Autodesk Fusion 360 part; units mm, degrees
(part 4 of 6)
  arc A493 (59.5878, 127.7864) -> (61.8532, 128.6962) centre (60.13, 129.7115) ccw
  arc A494 (58.8286, 130.1066) -> (59.5878, 127.7864) centre (60.7139, 129.4392) ccw
  arc A495 (58.8286, 130.1066) -> (58.5606, 130.7302) centre (58.3572, 130.2734) ccw
  line L124 (58.5606, 130.7302) -> (57.9668, 130.9946)
  arc A496 (57.9668, 130.9946) -> (57.324, 130.7764) centre (57.7634, 130.5378) ccw
  arc A497 (55.0918, 129.7882) -> (57.324, 130.7764) centre (55.5665, 131.731) ccw
  arc A498 (54.2521, 132.0804) -> (55.0918, 129.7882) centre (56.1596, 131.4793) ccw
  arc A499 (54.2521, 132.0804) -> (53.9625, 132.6943) centre (53.7752, 132.2307) ccw
  line L125 (53.9625, 132.6943) -> (53.3598, 132.9378)
  arc A500 (53.3598, 132.9378) -> (52.7251, 132.6974) centre (53.1725, 132.4742) ccw
  arc A501 (50.5287, 131.6318) -> (52.7251, 132.6974) centre (50.9353, 133.59) ccw
  arc A502 (49.6095, 133.8933) -> (50.5287, 131.6318) centre (51.5368, 133.3591) ccw
  arc A503 (49.6095, 133.8933) -> (49.2987, 134.4967) centre (49.1277, 134.0269) ccw
  line L126 (49.2987, 134.4967) -> (48.6879, 134.719)
  arc A504 (48.6879, 134.719) -> (48.0619, 134.4566) centre (48.5169, 134.2492) ccw
  arc A505 (45.904, 133.315) -> (48.0619, 134.4566) centre (46.2421, 135.2862) ccw
  arc A506 (44.9065, 135.5431) -> (45.904, 133.315) centre (46.8513, 135.0765) ccw
  arc A507 (44.9065, 135.5431) -> (44.5748, 136.1353) centre (44.4203, 135.6598) ccw
  line L127 (44.5748, 136.1353) -> (43.9566, 136.3362)
  arc A508 (43.9566, 136.3362) -> (43.3402, 136.052) centre (43.8021, 135.8606) ccw
  arc A509 (41.2235, 134.8358) -> (43.3402, 136.052) centre (41.4925, 136.8177) ccw
  arc A510 (40.1487, 137.0278) -> (41.2235, 134.8358) centre (42.1086, 136.6293) ccw
  arc A511 (40.1487, 137.0278) -> (39.7966, 137.608) centre (39.6587, 137.1274) ccw
  line L128 (39.7966, 137.608) -> (39.1717, 137.7872)
  arc A512 (39.1717, 137.7872) -> (38.5656, 137.4817) centre (39.0339, 137.3065) ccw
  arc A513 (36.4926, 136.1924) -> (38.5656, 137.4817) centre (36.6924, 138.1824) ccw
  arc A514 (35.3421, 138.3455) -> (36.4926, 136.1924) centre (37.3147, 138.0156) ccw
  arc A515 (35.3421, 138.3455) -> (34.9699, 138.9131) centre (34.8489, 138.4279) ccw
  line L129 (34.9699, 138.9131) -> (34.3392, 139.0703)
  arc A516 (34.3392, 139.0703) -> (33.7441, 138.7439) centre (34.2182, 138.5852) ccw
  arc A517 (31.7174, 137.383) -> (33.7441, 138.7439) centre (31.8475, 139.3787) ccw
  arc A518 (30.4923, 139.4946) -> (31.7174, 137.383) centre (32.4753, 139.2338) ccw
  arc A519 (30.4923, 139.4946) -> (30.1006, 140.0489) centre (29.9966, 139.5598) ccw
  line L130 (30.1006, 140.0489) -> (29.4648, 140.184)
  arc A520 (29.4648, 140.184) -> (28.8814, 139.837) centre (29.3608, 139.6949) ccw
  arc A521 (26.9034, 138.4062) -> (28.8814, 139.837) centre (26.9639, 140.4053) ccw
  arc A522 (25.6055, 140.4738) -> (26.9034, 138.4062) centre (27.5963, 140.2824) ccw
  arc A523 (25.6055, 140.4738) -> (25.1946, 141.014) centre (25.1078, 140.5216) ccw
  line L131 (25.1946, 141.014) -> (24.5545, 141.1269)
  arc A524 (24.5545, 141.1269) -> (23.9836, 140.7598) centre (24.4676, 140.6345) ccw
  arc A525 (22.0567, 139.2608) -> (23.9836, 140.7598) centre (22.0474, 141.2608) ccw
  arc A526 (20.6874, 141.2818) -> (22.0567, 139.2608) centre (22.6837, 141.16) ccw
  arc A527 (20.6874, 141.2818) -> (20.2579, 141.8074) centre (20.1883, 141.3123) ccw
  line L132 (20.2579, 141.8074) -> (19.6143, 141.8979)
  arc A528 (19.6143, 141.8979) -> (19.0565, 141.511) centre (19.5447, 141.4028) ccw
  arc A529 (17.1832, 139.9458) -> (19.0565, 141.511) centre (17.104, 141.9442) ccw
  arc A530 (15.7441, 141.9177) -> (17.1832, 139.9458) centre (17.7435, 141.8657) ccw
  arc A531 (15.7441, 141.9177) -> (15.2966, 142.428) centre (15.2443, 141.9308) ccw
  line L133 (15.2966, 142.428) -> (14.6501, 142.496)
  arc A532 (14.6501, 142.496) -> (14.1063, 142.0899) centre (14.5979, 141.9987) ccw
  arc A533 (12.2887, 140.4602) -> (14.1063, 142.0899) centre (12.1398, 142.4546) ccw
  arc A534 (10.7817, 142.3808) -> (12.2887, 140.4602) centre (12.7816, 142.3985) ccw
  arc A535 (10.7817, 142.3808) -> (10.3166, 142.8751) centre (10.2817, 142.3763) ccw
  line L134 (10.3166, 142.8751) -> (9.6682, 142.9205)
  arc A536 (9.6682, 142.9205) -> (9.1388, 142.4956) centre (9.6333, 142.4217) ccw
  arc A537 (7.3792, 140.8035) -> (9.1388, 142.4956) centre (7.1608, 142.7915) ccw
  arc A538 (5.8061, 142.6703) -> (7.3792, 140.8035) centre (7.8042, 142.7578) ccw
  arc A539 (5.8061, 142.6703) -> (5.324, 143.1481) centre (5.3066, 142.6484) ccw
  line L135 (5.324, 143.1481) -> (4.6744, 143.1708)
  arc A540 (4.6744, 143.1708) -> (4.1602, 142.7278) centre (4.657, 142.6711) ccw
  arc A541 (2.4607, 140.9752) -> (4.1602, 142.7278) centre (2.1731, 142.9545) ccw
  arc A542 (0.8235, 142.786) -> (2.4607, 140.9752) centre (2.8173, 142.9432) ccw
  arc A543 (0.8235, 142.786) -> (0.325, 143.2467) centre (0.325, 142.7467) ccw
  line L136 (0.325, 143.2467) -> (-0.325, 143.2467)
  arc A544 (-0.325, 143.2467) -> (-0.8235, 142.786) centre (-0.325, 142.7467) ccw
  arc A545 (-2.4607, 140.9752) -> (-0.8235, 142.786) centre (-2.8173, 142.9432) ccw
  arc A546 (-4.1602, 142.7278) -> (-2.4607, 140.9752) centre (-2.1731, 142.9545) ccw
  arc A547 (-4.1602, 142.7278) -> (-4.6744, 143.1708) centre (-4.657, 142.6711) ccw
  line L137 (-4.6744, 143.1708) -> (-5.324, 143.1481)
  arc A548 (-5.324, 143.1481) -> (-5.8061, 142.6703) centre (-5.3066, 142.6484) ccw
  arc A549 (-7.3792, 140.8035) -> (-5.8061, 142.6703) centre (-7.8042, 142.7578) ccw
  arc A550 (-9.1388, 142.4956) -> (-7.3792, 140.8035) centre (-7.1608, 142.7915) ccw
  arc A551 (-9.1388, 142.4956) -> (-9.6682, 142.9205) centre (-9.6333, 142.4217) ccw
  line L138 (-9.6682, 142.9205) -> (-10.3166, 142.8751)
  arc A552 (-10.3166, 142.8751) -> (-10.7817, 142.3808) centre (-10.2817, 142.3763) ccw
  arc A553 (-12.2887, 140.4602) -> (-10.7817, 142.3808) centre (-12.7816, 142.3985) ccw
  arc A554 (-14.1063, 142.0899) -> (-12.2887, 140.4602) centre (-12.1398, 142.4546) ccw
  arc A555 (-14.1063, 142.0899) -> (-14.6501, 142.496) centre (-14.5979, 141.9987) ccw
  line L139 (-14.6501, 142.496) -> (-15.2966, 142.428)
  arc A556 (-15.2966, 142.428) -> (-15.7441, 141.9177) centre (-15.2443, 141.9308) ccw
  arc A557 (-17.1832, 139.9458) -> (-15.7441, 141.9177) centre (-17.7435, 141.8657) ccw
  arc A558 (-19.0565, 141.511) -> (-17.1832, 139.9458) centre (-17.104, 141.9442) ccw
  arc A559 (-19.0565, 141.511) -> (-19.6143, 141.8979) centre (-19.5447, 141.4028) ccw
  line L140 (-19.6143, 141.8979) -> (-20.2579, 141.8074)
  arc A560 (-20.2579, 141.8074) -> (-20.6874, 141.2818) centre (-20.1883, 141.3123) ccw
  arc A561 (-22.0567, 139.2608) -> (-20.6874, 141.2818) centre (-22.6837, 141.16) ccw
  arc A562 (-23.9836, 140.7598) -> (-22.0567, 139.2608) centre (-22.0474, 141.2608) ccw
  arc A563 (-23.9836, 140.7598) -> (-24.5545, 141.1269) centre (-24.4676, 140.6345) ccw
  line L141 (-24.5545, 141.1269) -> (-25.1946, 141.014)
  arc A564 (-25.1946, 141.014) -> (-25.6055, 140.4738) centre (-25.1078, 140.5216) ccw
  arc A565 (-26.9034, 138.4062) -> (-25.6055, 140.4738) centre (-27.5963, 140.2824) ccw
  arc A566 (-28.8814, 139.837) -> (-26.9034, 138.4062) centre (-26.9639, 140.4053) ccw
  arc A567 (-28.8814, 139.837) -> (-29.4648, 140.184) centre (-29.3608, 139.6949) ccw
  line L142 (-29.4648, 140.184) -> (-30.1006, 140.0489)
  arc A568 (-30.1006, 140.0489) -> (-30.4923, 139.4946) centre (-29.9966, 139.5598) ccw
  arc A569 (-31.7174, 137.383) -> (-30.4923, 139.4946) centre (-32.4753, 139.2338) ccw
  arc A570 (-33.7441, 138.7439) -> (-31.7174, 137.383) centre (-31.8475, 139.3787) ccw
  arc A571 (-33.7441, 138.7439) -> (-34.3392, 139.0703) centre (-34.2182, 138.5852) ccw
  line L143 (-34.3392, 139.0703) -> (-34.9699, 138.9131)
  arc A572 (-34.9699, 138.9131) -> (-35.3421, 138.3455) centre (-34.8489, 138.4279) ccw
  arc A573 (-36.4926, 136.1924) -> (-35.3421, 138.3455) centre (-37.3147, 138.0156) ccw
  arc A574 (-38.5656, 137.4817) -> (-36.4926, 136.1924) centre (-36.6924, 138.1824) ccw
  arc A575 (-38.5656, 137.4817) -> (-39.1717, 137.7872) centre (-39.0339, 137.3065) ccw
  line L144 (-39.1717, 137.7872) -> (-39.7966, 137.608)
  arc A576 (-39.7966, 137.608) -> (-40.1487, 137.0278) centre (-39.6587, 137.1274) ccw
  arc A577 (-41.2235, 134.8358) -> (-40.1487, 137.0278) centre (-42.1086, 136.6293) ccw
  arc A578 (-43.3402, 136.052) -> (-41.2235, 134.8358) centre (-41.4925, 136.8177) ccw
  arc A579 (-43.3402, 136.052) -> (-43.9566, 136.3362) centre (-43.8021, 135.8606) ccw
  line L145 (-43.9566, 136.3362) -> (-44.5748, 136.1353)
  arc A580 (-44.5748, 136.1353) -> (-44.9065, 135.5431) centre (-44.4203, 135.6598) ccw
  arc A581 (-45.904, 133.315) -> (-44.9065, 135.5431) centre (-46.8513, 135.0765) ccw
  arc A582 (-48.0619, 134.4566) -> (-45.904, 133.315) centre (-46.2421, 135.2862) ccw
  arc A583 (-48.0619, 134.4566) -> (-48.6879, 134.719) centre (-48.5169, 134.2492) ccw
  line L146 (-48.6879, 134.719) -> (-49.2987, 134.4967)
  arc A584 (-49.2987, 134.4967) -> (-49.6095, 133.8933) centre (-49.1277, 134.0269) ccw
  arc A585 (-50.5287, 131.6318) -> (-49.6095, 133.8933) centre (-51.5368, 133.3591) ccw
  arc A586 (-52.7251, 132.6974) -> (-50.5287, 131.6318) centre (-50.9353, 133.59) ccw
  arc A587 (-52.7251, 132.6974) -> (-53.3598, 132.9378) centre (-53.1725, 132.4742) ccw
  line L147 (-53.3598, 132.9378) -> (-53.9625, 132.6943)
  arc A588 (-53.9625, 132.6943) -> (-54.2521, 132.0804) centre (-53.7752, 132.2307) ccw
  arc A589 (-55.0918, 129.7882) -> (-54.2521, 132.0804) centre (-56.1596, 131.4793) ccw
  arc A590 (-57.324, 130.7764) -> (-55.0918, 129.7882) centre (-55.5665, 131.731) ccw
  arc A591 (-57.324, 130.7764) -> (-57.9668, 130.9946) centre (-57.7634, 130.5378) ccw
  line L148 (-57.9668, 130.9946) -> (-58.5606, 130.7302)
  arc A592 (-58.5606, 130.7302) -> (-58.8286, 130.1066) centre (-58.3572, 130.2734) ccw
  arc A593 (-59.5878, 127.7864) -> (-58.8286, 130.1066) centre (-60.7139, 129.4392) ccw
  arc A594 (-61.8532, 128.6962) -> (-59.5878, 127.7864) centre (-60.13, 129.7115) ccw
  arc A595 (-61.8532, 128.6962) -> (-62.5031, 128.8918) centre (-62.2839, 128.4424) ccw
  line L149 (-62.5031, 128.8918) -> (-63.0873, 128.6068)
  arc A596 (-63.0873, 128.6068) -> (-63.3334, 127.9742) centre (-62.8682, 128.1574) ccw
  arc A597 (-64.0112, 125.629) -> (-63.3334, 127.9742) centre (-65.1943, 127.2415) ccw
  arc A598 (-66.3069, 126.4592) -> (-64.0112, 125.629) centre (-64.6203, 127.534) ccw
  arc A599 (-66.3069, 126.4592) -> (-66.9633, 126.6319) centre (-66.7286, 126.1905) ccw
  line L150 (-66.9633, 126.6319) -> (-67.5372, 126.3268)
  arc A600 (-67.5372, 126.3268) -> (-67.761, 125.686) centre (-67.3025, 125.8853) ccw
  arc A601 (-68.3566, 123.3185) -> (-67.761, 125.686) centre (-69.5953, 124.8887) ccw
  arc A602 (-70.6799, 124.068) -> (-68.3566, 123.3185) centre (-69.0318, 125.2011) ccw
  arc A603 (-70.6799, 124.068) -> (-71.3419, 124.2178) centre (-71.0919, 123.7848) ccw
  line L151 (-71.3419, 124.2178) -> (-71.9048, 123.8928)
  arc A604 (-71.9048, 123.8928) -> (-72.1061, 123.2446) centre (-71.6548, 123.4598) ccw
  arc A605 (-72.6187, 120.8578) -> (-72.1061, 123.2446) centre (-73.9114, 122.3838) ccw
  arc A606 (-74.9667, 121.5258) -> (-72.6187, 120.8578) centre (-73.3592, 122.7156) ccw
  arc A607 (-74.9667, 121.5258) -> (-75.6336, 121.6523) centre (-75.3686, 121.2283) ccw
  line L152 (-75.6336, 121.6523) -> (-76.1848, 121.3079)
  arc A608 (-76.1848, 121.3079) -> (-76.3634, 120.653) centre (-75.9199, 120.8839) ccw
  arc A609 (-76.7923, 118.2498) -> (-76.3634, 120.653) centre (-78.1375, 119.7298) ccw
  arc A610 (-79.1623, 118.8354) -> (-76.7923, 118.2498) centre (-77.5972, 120.0807) ccw
  arc A611 (-79.1623, 118.8354) -> (-79.8331, 118.9387) centre (-79.5535, 118.5241) ccw
  line L153 (-79.8331, 118.9387) -> (-80.372, 118.5752)
  arc A612 (-80.372, 118.5752) -> (-80.5276, 117.9145) centre (-80.0924, 118.1607) ccw
  arc A613 (-80.8724, 115.4978) -> (-80.5276, 117.9145) centre (-82.2684, 116.9299) ccw
  arc A614 (-83.2613, 116.0003) -> (-80.8724, 115.4978) centre (-81.7407, 117.2994) ccw
  arc A615 (-83.2613, 116.0003) -> (-83.9354, 116.0801) centre (-83.6415, 115.6756) ccw
  line L154 (-83.9354, 116.0801) -> (-84.4612, 115.698)
  arc A616 (-84.4612, 115.698) -> (-84.5937, 115.0323) centre (-84.1673, 115.2935) ccw
  arc A617 (-84.8539, 112.605) -> (-84.5937, 115.0323) centre (-86.2991, 113.9875) ccw
  arc A618 (-87.259, 113.0239) -> (-84.8539, 112.605) centre (-85.7846, 114.3753) ccw
  arc A619 (-87.259, 113.0239) -> (-87.9354, 113.08) centre (-87.6276, 112.686) ccw
  line L155 (-87.9354, 113.08) -> (-88.4476, 112.6799)
  arc A620 (-88.4476, 112.6799) -> (-88.5567, 112.01) centre (-88.1398, 112.2859) ccw
  arc A621 (-88.7321, 109.575) -> (-88.5567, 112.01) centre (-90.2247, 110.9063) ccw
  arc A622 (-91.1503, 109.9097) -> (-88.7321, 109.575) centre (-89.724, 111.3118) ccw
  arc A623 (-91.1503, 109.9097) -> (-91.8283, 109.9423) centre (-91.5069, 109.5592) ccw
  line L156 (-91.8283, 109.9423) -> (-92.3262, 109.5244)
  arc A624 (-92.3262, 109.5244) -> (-92.4119, 108.8511) centre (-92.0048, 109.1414) ccw
  arc A625 (-92.5022, 106.4116) -> (-92.4119, 108.8511) centre (-94.0403, 107.6899) ccw
  arc A626 (-94.9306, 106.6617) -> (-92.5022, 106.4116) centre (-93.554, 108.1126) ccw
  arc A627 (-94.9306, 106.6617) -> (-95.6092, 106.6705) centre (-95.2747, 106.299) ccw
  line L157 (-95.6092, 106.6705) -> (-96.0923, 106.2356)
  arc A628 (-96.0923, 106.2356) -> (-96.1544, 105.5597) centre (-95.7577, 105.864) ccw
  arc A629 (-96.1595, 103.1185) -> (-96.1544, 105.5597) centre (-97.7413, 104.3424) ccw
  arc A630 (-98.5952, 103.2837) -> (-96.1595, 103.1185) centre (-97.2701, 104.7818) ccw
  arc A631 (-98.5952, 103.2837) -> (-99.2737, 103.2688) centre (-98.9264, 102.9092) ccw
  line L158 (-99.2737, 103.2688) -> (-99.7413, 102.8173)
  arc A632 (-99.7413, 102.8173) -> (-99.7798, 102.1396) centre (-99.394, 102.4576) ccw
  arc A633 (-99.6997, 99.6997) -> (-99.7798, 102.1396) centre (-101.3233, 100.8677) ccw
  arc A634 (-102.1396, 99.7798) -> (-99.6997, 99.6997) centre (-100.8677, 101.3233) ccw
  arc A635 (-102.1396, 99.7798) -> (-102.8173, 99.7413) centre (-102.4576, 99.394) ccw
  line L159 (-102.8173, 99.7413) -> (-103.2688, 99.2737)
  arc A636 (-103.2688, 99.2737) -> (-103.2837, 98.5952) centre (-102.9092, 98.9264) ccw
  arc A637 (-103.1185, 96.1595) -> (-103.2837, 98.5952) centre (-104.7818, 97.2701) ccw
  arc A638 (-105.5597, 96.1544) -> (-103.1185, 96.1595) centre (-104.3424, 97.7413) ccw
  arc A639 (-105.5597, 96.1544) -> (-106.2356, 96.0923) centre (-105.864, 95.7577) ccw
  line L160 (-106.2356, 96.0923) -> (-106.6705, 95.6092)
  arc A640 (-106.6705, 95.6092) -> (-106.6617, 94.9306) centre (-106.299, 95.2747) ccw
  arc A641 (-106.4116, 92.5022) -> (-106.6617, 94.9306) centre (-108.1126, 93.554) ccw
  arc A642 (-108.8511, 92.4119) -> (-106.4116, 92.5022) centre (-107.6899, 94.0403) ccw
  arc A643 (-108.8511, 92.4119) -> (-109.5244, 92.3262) centre (-109.1414, 92.0048) ccw
  line L161 (-109.5244, 92.3262) -> (-109.9423, 91.8283)
  arc A644 (-109.9423, 91.8283) -> (-109.9097, 91.1503) centre (-109.5592, 91.5069) ccw
  arc A645 (-109.575, 88.7321) -> (-109.9097, 91.1503) centre (-111.3118, 89.724) ccw
  arc A646 (-112.01, 88.5567) -> (-109.575, 88.7321) centre (-110.9063, 90.2247) ccw
  arc A647 (-112.01, 88.5567) -> (-112.6799, 88.4476) centre (-112.2859, 88.1398) ccw
  line L162 (-112.6799, 88.4476) -> (-113.08, 87.9354)
  arc A648 (-113.08, 87.9354) -> (-113.0239, 87.259) centre (-112.686, 87.6276) ccw
  arc A649 (-112.605, 84.8539) -> (-113.0239, 87.259) centre (-114.3753, 85.7846) ccw
  arc A650 (-115.0323, 84.5937) -> (-112.605, 84.8539) centre (-113.9875, 86.2991) ccw
  arc A651 (-115.0323, 84.5937) -> (-115.698, 84.4612) centre (-115.2935, 84.1673) ccw
  line L163 (-115.698, 84.4612) -> (-116.0801, 83.9354)
  arc A652 (-116.0801, 83.9354) -> (-116.0003, 83.2613) centre (-115.6756, 83.6415) ccw
  arc A653 (-115.4978, 80.8724) -> (-116.0003, 83.2613) centre (-117.2994, 81.7407) ccw
  arc A654 (-117.9145, 80.5276) -> (-115.4978, 80.8724) centre (-116.9299, 82.2684) ccw
  arc A655 (-117.9145, 80.5276) -> (-118.5752, 80.372) centre (-118.1607, 80.0924) ccw
  line L164 (-118.5752, 80.372) -> (-118.9387, 79.8331)
  arc A656 (-118.9387, 79.8331) -> (-118.8354, 79.1623) centre (-118.5241, 79.5535) ccw
  arc A657 (-118.2498, 76.7923) -> (-118.8354, 79.1623) centre (-120.0807, 77.5972) ccw
  arc A658 (-120.653, 76.3634) -> (-118.2498, 76.7923) centre (-119.7298, 78.1375) ccw
  arc A659 (-120.653, 76.3634) -> (-121.3079, 76.1848) centre (-120.8839, 75.9199) ccw
  line L165 (-121.3079, 76.1848) -> (-121.6523, 75.6336)
  arc A660 (-121.6523, 75.6336) -> (-121.5258, 74.9667) centre (-121.2283, 75.3686) ccw
  arc A661 (-120.8578, 72.6187) -> (-121.5258, 74.9667) centre (-122.7156, 73.3592) ccw
  arc A662 (-123.2446, 72.1061) -> (-120.8578, 72.6187) centre (-122.3838, 73.9114) ccw
  arc A663 (-123.2446, 72.1061) -> (-123.8928, 71.9048) centre (-123.4598, 71.6548) ccw
  line L166 (-123.8928, 71.9048) -> (-124.2178, 71.3419)
  arc A664 (-124.2178, 71.3419) -> (-124.068, 70.6799) centre (-123.7848, 71.0919) ccw
  arc A665 (-123.3185, 68.3566) -> (-124.068, 70.6799) centre (-125.2011, 69.0318) ccw
  arc A666 (-125.686, 67.761) -> (-123.3185, 68.3566) centre (-124.8887, 69.5953) ccw
  arc A667 (-125.686, 67.761) -> (-126.3268, 67.5372) centre (-125.8853, 67.3025) ccw
  line L167 (-126.3268, 67.5372) -> (-126.6319, 66.9633)
  arc A668 (-126.6319, 66.9633) -> (-126.4592, 66.3069) centre (-126.1905, 66.7286) ccw
  arc A669 (-125.629, 64.0112) -> (-126.4592, 66.3069) centre (-127.534, 64.6203) ccw
  arc A670 (-127.9742, 63.3334) -> (-125.629, 64.0112) centre (-127.2415, 65.1943) ccw
  arc A671 (-127.9742, 63.3334) -> (-128.6068, 63.0873) centre (-128.1574, 62.8682) ccw
  line L168 (-128.6068, 63.0873) -> (-128.8918, 62.5031)
  arc A672 (-128.8918, 62.5031) -> (-128.6962, 61.8532) centre (-128.4424, 62.2839) ccw
  arc A673 (-127.7864, 59.5878) -> (-128.6962, 61.8532) centre (-129.7115, 60.13) ccw
  arc A674 (-130.1066, 58.8286) -> (-127.7864, 59.5878) centre (-129.4392, 60.7139) ccw
  arc A675 (-130.1066, 58.8286) -> (-130.7302, 58.5606) centre (-130.2734, 58.3572) ccw
  line L169 (-130.7302, 58.5606) -> (-130.9946, 57.9668)
  arc A676 (-130.9946, 57.9668) -> (-130.7764, 57.324) centre (-130.5378, 57.7634) ccw
  arc A677 (-129.7882, 55.0918) -> (-130.7764, 57.324) centre (-131.731, 55.5665) ccw
  arc A678 (-132.0804, 54.2521) -> (-129.7882, 55.0918) centre (-131.4793, 56.1596) ccw
  arc A679 (-132.0804, 54.2521) -> (-132.6943, 53.9625) centre (-132.2307, 53.7752) ccw
  line L170 (-132.6943, 53.9625) -> (-132.9378, 53.3598)
  arc A680 (-132.9378, 53.3598) -> (-132.6974, 52.7251) centre (-132.4742, 53.1725) ccw
  arc A681 (-131.6318, 50.5287) -> (-132.6974, 52.7251) centre (-133.59, 50.9353) ccw
  arc A682 (-133.8933, 49.6095) -> (-131.6318, 50.5287) centre (-133.3591, 51.5368) ccw
  arc A683 (-133.8933, 49.6095) -> (-134.4967, 49.2987) centre (-134.0269, 49.1277) ccw
  line L171 (-134.4967, 49.2987) -> (-134.719, 48.6879)
  arc A684 (-134.719, 48.6879) -> (-134.4566, 48.0619) centre (-134.2492, 48.5169) ccw
  arc A685 (-133.315, 45.904) -> (-134.4566, 48.0619) centre (-135.2862, 46.2421) ccw
  arc A686 (-135.5431, 44.9065) -> (-133.315, 45.904) centre (-135.0765, 46.8513) ccw
  arc A687 (-135.5431, 44.9065) -> (-136.1353, 44.5748) centre (-135.6598, 44.4203) ccw
  line L172 (-136.1353, 44.5748) -> (-136.3362, 43.9566)
  arc A688 (-136.3362, 43.9566) -> (-136.052, 43.3402) centre (-135.8606, 43.8021) ccw
  arc A689 (-134.8358, 41.2235) -> (-136.052, 43.3402) centre (-136.8177, 41.4925) ccw
  arc A690 (-137.0278, 40.1487) -> (-134.8358, 41.2235) centre (-136.6293, 42.1086) ccw
  arc A691 (-137.0278, 40.1487) -> (-137.608, 39.7966) centre (-137.1274, 39.6587) ccw
  line L173 (-137.608, 39.7966) -> (-137.7872, 39.1717)
  arc A692 (-137.7872, 39.1717) -> (-137.4817, 38.5656) centre (-137.3065, 39.0339) ccw
  arc A693 (-136.1924, 36.4926) -> (-137.4817, 38.5656) centre (-138.1824, 36.6924) ccw
  arc A694 (-138.3455, 35.3421) -> (-136.1924, 36.4926) centre (-138.0156, 37.3147) ccw
  arc A695 (-138.3455, 35.3421) -> (-138.9131, 34.9699) centre (-138.4279, 34.8489) ccw
  line L174 (-138.9131, 34.9699) -> (-139.0703, 34.3392)
  arc A696 (-139.0703, 34.3392) -> (-138.7439, 33.7441) centre (-138.5852, 34.2182) ccw
  arc A697 (-137.383, 31.7174) -> (-138.7439, 33.7441) centre (-139.3787, 31.8475) ccw
  arc A698 (-139.4946, 30.4923) -> (-137.383, 31.7174) centre (-139.2338, 32.4753) ccw
  arc A699 (-139.4946, 30.4923) -> (-140.0489, 30.1006) centre (-139.5598, 29.9966) ccw
  line L175 (-140.0489, 30.1006) -> (-140.184, 29.4648)
  arc A700 (-140.184, 29.4648) -> (-139.837, 28.8814) centre (-139.6949, 29.3608) ccw
  arc A701 (-138.4062, 26.9034) -> (-139.837, 28.8814) centre (-140.4053, 26.9639) ccw
  arc A702 (-140.4738, 25.6055) -> (-138.4062, 26.9034) centre (-140.2824, 27.5963) ccw
  arc A703 (-140.4738, 25.6055) -> (-141.014, 25.1946) centre (-140.5216, 25.1078) ccw
  line L176 (-141.014, 25.1946) -> (-141.1269, 24.5545)
  arc A704 (-141.1269, 24.5545) -> (-140.7598, 23.9836) centre (-140.6345, 24.4676) ccw
  arc A705 (-139.2608, 22.0567) -> (-140.7598, 23.9836) centre (-141.2608, 22.0474) ccw
  arc A706 (-141.2818, 20.6874) -> (-139.2608, 22.0567) centre (-141.16, 22.6837) ccw
  arc A707 (-141.2818, 20.6874) -> (-141.8074, 20.2579) centre (-141.3123, 20.1883) ccw
  line L177 (-141.8074, 20.2579) -> (-141.8979, 19.6143)
  arc A708 (-141.8979, 19.6143) -> (-141.511, 19.0565) centre (-141.4028, 19.5447) ccw
  arc A709 (-139.9458, 17.1832) -> (-141.511, 19.0565) centre (-141.9442, 17.104) ccw
  arc A710 (-141.9177, 15.7441) -> (-139.9458, 17.1832) centre (-141.8657, 17.7435) ccw
  arc A711 (-141.9177, 15.7441) -> (-142.428, 15.2966) centre (-141.9308, 15.2443) ccw
  line L178 (-142.428, 15.2966) -> (-142.496, 14.6501)
  arc A712 (-142.496, 14.6501) -> (-142.0899, 14.1063) centre (-141.9987, 14.5979) ccw
  arc A713 (-140.4602, 12.2887) -> (-142.0899, 14.1063) centre (-142.4546, 12.1398) ccw
  arc A714 (-142.3808, 10.7817) -> (-140.4602, 12.2887) centre (-142.3985, 12.7816) ccw
  arc A715 (-142.3808, 10.7817) -> (-142.8751, 10.3166) centre (-142.3763, 10.2817) ccw
  line L179 (-142.8751, 10.3166) -> (-142.9205, 9.6682)
  arc A716 (-142.9205, 9.6682) -> (-142.4956, 9.1388) centre (-142.4217, 9.6333) ccw
  arc A717 (-140.8035, 7.3792) -> (-142.4956, 9.1388) centre (-142.7915, 7.1608) ccw
  arc A718 (-142.6703, 5.8061) -> (-140.8035, 7.3792) centre (-142.7578, 7.8042) ccw
  arc A719 (-142.6703, 5.8061) -> (-143.1481, 5.324) centre (-142.6484, 5.3066) ccw
  circle A720 centre (0, 0) radius 145
  dimension "d12" = 290
  constraint coincident A720.centre origin
  measures "d12" diameter of A720
extrude "Extrude2" add sketch "Sketch2" along normal blind 2 contours L0 A0 A1 A2 A3 L1 A4 A5 A6 A7 L2 A8 A9 A10 A11 L3 A12 A13 A14 A15 L4 A16 A17 A18 A19 L5 A20 A21 A22 A23 L6 A24 A25 A26 A27 L7 A28 A29 A30 A31 L8 A32 A33 A34 A35 L9 A36 A37 A38 A39 L10 A40 A41 A42 A43 L11 A44 A45 A46 A47 L12 A48 A49 A50 A51 L13 A52 A53 A54 A55 L14 A56 A57 A58 A59 L15 A60 A61 A62 A63 L16 A64 A65 A66 A67 L17 A68 A69 A70 A71 L18 A72 A73 A74 A75 L19 A76 A77 A78 A79 L20 A80 A81 A82 A83 L21 A84 A85 A86 A87 L22 A88 A89 A90 A91 L23 A92 A93 A94 A95 L24 A96 A97 A98 A99 L25 A100 A101 A102 A103 L26 A104 A105 A106 A107 L27 A108 A109 A110 A111 L28 A112 A113 A114 A115 L29 A116 A117 A118 A119 L30 A120 A121 A122 A123 L31 A124 A125 A126 A127 L32 A128 A129 A130 A131 L33 A132 A133 A134 A135 L34 A136 A137 A138 A139 L35 A140 A141 A142 A143 L36 A144 A145 A146 A147 L37 A148 A149 A150 A151 L38 A152 A153 A154 A155 L39 A156 A157 A158 A159 L40 A160 A161 A162 A163 L41 A164 A165 A166 A167 L42 A168 A169 A170 A171 L43 A172 A173 A174 A175 L44 A176 A177 A178 A179 L45 A180 A181 A182 A183 L46 A184 A185 A186 A187 L47 A188 A189 A190 A191 L48 A192 A193 A194 A195 L49 A196 A197 A198 A199 L50 A200 A201 A202 A203 L51 A204 A205 A206 A207 L52 A208 A209 A210 A211 L53 A212 A213 A214 A215 L54 A216 A217 A218 A219 L55 A220 A221 A222 A223 L56 A224 A225 A226 A227 L57 A228 A229 A230 A231 L58 A232 A233 A234 A235 L59 A236 A237 A238 A239 L60 A240 A241 A242 A243 L61 A244 A245 A246 A247 L62 A248 A249 A250 A251 L63 A252 A253 A254 A255 L64 A256 A257 A258 A259 L65 A260 A261 A262 A263 L66 A264 A265 A266 A267 L67 A268 A269 A270 A271 L68 A272 A273 A274 A275 L69 A276 A277 A278 A279 L70 A280 A281 A282 A283 L71 A284 A285 A286 A287 L72 A288 A289 A290 A291 L73 A292 A293 A294 A295 L74 A296 A297 A298 A299 L75 A300 A301 A302 A303 L76 A304 A305 A306 A307 L77 A308 A309 A310 A311 L78 A312 A313 A314 A315 L79 A316 A317 A318 A319 L80 A320 A321 A322 A323 L81 A324 A325 A326 A327 L82 A328 A329 A330 A331 L83 A332 A333 A334 A335 L84 A336 A337 A338 A339 L85 A340 A341 A342 A343 L86 A344 A345 A346 A347 L87 A348 A349 A350 A351 L88 A352 A353 A354 A355 L89 A356 A357 A358 A359 L90 A360 A361 A362 A363 L91 A364 A365 A366 A367 L92 A368 A369 A370 A371 L93 A372 A373 A374 A375 L94 A376 A377 A378 A379 L95 A380 A381 A382 A383 L96 A384 A385 A386 A387 L97 A388 A389 A390 A391 L98 A392 A393 A394 A395 L99 A396 A397 A398 A399 L100 A400 A401 A402 A403 L101 A404 A405 A406 A407 L102 A408 A409 A410 A411 L103 A412 A413 A414 A415 L104 A416 A417 A418 A419 L105 A420 A421 A422 A423 L106 A424 A425 A426 A427 L107 A428 A429 A430 A431 L108 A432 A433 A434 A435 L109 A436 A437 A438 A439 L110 A440 A441 A442 A443 L111 A444 A445 A446 A447 L112 A448 A449 A450 A451 L113 A452 A453 A454 A455 L114 A456 A457 A458 A459 L115 A460 A461 A462 A463 L116 A464 A465 A466 A467 L117 A468 A469 A470 A471 L118 A472 A473 A474 A475 L119 A476 A477 A478 A479 L120 A480 A481 A482 A483 L121 A484 A485 A486 A487 L122 A488 A489 A490 A491 L123 A492 A493 A494 A495 L124 A496 A497 A498 A499 L125 A500 A501 A502 A503 L126 A504 A505 A506 A507 L127 A508 A509 A510 A511 L128 A512 A513 A514 A515 L129 A516 A517 A518 A519 L130 A520 A521 A522 A523 L131 A524 A525 A526 A527 L132 A528 A529 A530 A531 L133 A532 A533 A534 A535 L134 A536 A537 A538 A539 L135 A540 A541 A542 A543 L136 A544 A545 A546 A547 L137 A548 A549 A550 A551 L138 A552 A553 A554 A555 L139 A556 A557 A558 A559 L140 A560 A561 A562 A563 L141 A564 A565 A566 A567 L142 A568 A569 A570 A571 L143 A572 A573 A574 A575 L144 A576 A577 A578 A579 L145 A580 A581 A582 A583 L146 A584 A585 A586 A587 L147 A588 A589 A590 A591 L148 A592 A593 A594 A595 L149 A596 A597 A598 A599 L150 A600 A601 A602 A603 L151 A604 A605 A606 A607 L152 A608 A609 A610 A611 L153 A612 A613 A614 A615 L154 A616 A617 A618 A619 L155 A620 A621 A622 A623 L156 A624 A625 A626 A627 L157 A628 A629 A630 A631 L158 A632 A633 A634 A635 L159 A636 A637 A638 A639 L160 A640 A641 A642 A643 L161 A644 A645 A646 A647 L162 A648 A649 A650 A651 L163 A652 A653 A654 A655 L164 A656 A657 A658 A659 L165 A660 A661 A662 A663 L166 A664 A665 A666 A667 L167 A668 A669 A670 A671 L168 A672 A673 A674 A675 L169 A676 A677 A678 A679 L170 A680 A681 A682 A683 L171 A684 A685 A686 A687 L172 A688 A689 A690 A691 L173 A692 A693 A694 A695 L174 A696 A697 A698 A699 L175 A700 A701 A702 A703 L176 A704 A705 A706 A707 L177 A708 A709 A710 A711 L178 A712 A713 A714 A715 L179 A716 A717 A718 A719 | A720
sketch "Sketch3" plane through (0, 0, 0) normal (0, 0, -1) x (1, 0, 0)
  line L0 (143.1708, 4.6744) -> (143.1481, 5.324)
  arc A0 (143.1481, 5.324) -> (142.6703, 5.8061) centre (142.6484, 5.3066) ccw
  arc A1 (140.8035, 7.3792) -> (142.6703, 5.8061) centre (142.7578, 7.8042) ccw
  arc A2 (142.4956, 9.1388) -> (140.8035, 7.3792) centre (142.7915, 7.1608) ccw
  arc A3 (142.4956, 9.1388) -> (142.9205, 9.6682) centre (142.4217, 9.6333) ccw
  line L1 (142.9205, 9.6682) -> (142.8751, 10.3166)
  arc A4 (142.8751, 10.3166) -> (142.3808, 10.7817) centre (142.3763, 10.2817) ccw
  arc A5 (140.4602, 12.2887) -> (142.3808, 10.7817) centre (142.3985, 12.7816) ccw
  arc A6 (142.0899, 14.1063) -> (140.4602, 12.2887) centre (142.4546, 12.1398) ccw
  arc A7 (142.0899, 14.1063) -> (142.496, 14.6501) centre (141.9987, 14.5979) ccw
  line L2 (142.496, 14.6501) -> (142.428, 15.2966)
  arc A8 (142.428, 15.2966) -> (141.9177, 15.7441) centre (141.9308, 15.2443) ccw
  arc A9 (139.9458, 17.1832) -> (141.9177, 15.7441) centre (141.8657, 17.7435) ccw
  arc A10 (141.511, 19.0565) -> (139.9458, 17.1832) centre (141.9442, 17.104) ccw
  arc A11 (141.511, 19.0565) -> (141.8979, 19.6143) centre (141.4028, 19.5447) ccw
  line L3 (141.8979, 19.6143) -> (141.8074, 20.2579)
  arc A12 (141.8074, 20.2579) -> (141.2818, 20.6874) centre (141.3123, 20.1883) ccw
  arc A13 (139.2608, 22.0567) -> (141.2818, 20.6874) centre (141.16, 22.6837) ccw
  arc A14 (140.7598, 23.9836) -> (139.2608, 22.0567) centre (141.2608, 22.0474) ccw
  arc A15 (140.7598, 23.9836) -> (141.1269, 24.5545) centre (140.6345, 24.4676) ccw
  line L4 (141.1269, 24.5545) -> (141.014, 25.1946)
  arc A16 (141.014, 25.1946) -> (140.4738, 25.6055) centre (140.5216, 25.1078) ccw
  arc A17 (138.4062, 26.9034) -> (140.4738, 25.6055) centre (140.2824, 27.5963) ccw
  arc A18 (139.837, 28.8814) -> (138.4062, 26.9034) centre (140.4053, 26.9639) ccw
  arc A19 (139.837, 28.8814) -> (140.184, 29.4648) centre (139.6949, 29.3608) ccw
  line L5 (140.184, 29.4648) -> (140.0489, 30.1006)
  arc A20 (140.0489, 30.1006) -> (139.4946, 30.4923) centre (139.5598, 29.9966) ccw
  arc A21 (137.383, 31.7174) -> (139.4946, 30.4923) centre (139.2338, 32.4753) ccw
  arc A22 (138.7439, 33.7441) -> (137.383, 31.7174) centre (139.3787, 31.8475) ccw
  arc A23 (138.7439, 33.7441) -> (139.0703, 34.3392) centre (138.5852, 34.2182) ccw
  line L6 (139.0703, 34.3392) -> (138.9131, 34.9699)
  arc A24 (138.9131, 34.9699) -> (138.3455, 35.3421) centre (138.4279, 34.8489) ccw
  arc A25 (136.1924, 36.4926) -> (138.3455, 35.3421) centre (138.0156, 37.3147) ccw
  arc A26 (137.4817, 38.5656) -> (136.1924, 36.4926) centre (138.1824, 36.6924) ccw
  arc A27 (137.4817, 38.5656) -> (137.7872, 39.1717) centre (137.3065, 39.0339) ccw
  line L7 (137.7872, 39.1717) -> (137.608, 39.7966)
  arc A28 (137.608, 39.7966) -> (137.0278, 40.1487) centre (137.1274, 39.6587) ccw
  arc A29 (134.8358, 41.2235) -> (137.0278, 40.1487) centre (136.6293, 42.1086) ccw
  arc A30 (136.052, 43.3402) -> (134.8358, 41.2235) centre (136.8177, 41.4925) ccw
  arc A31 (136.052, 43.3402) -> (136.3362, 43.9566) centre (135.8606, 43.8021) ccw
  line L8 (136.3362, 43.9566) -> (136.1353, 44.5748)
  arc A32 (136.1353, 44.5748) -> (135.5431, 44.9065) centre (135.6598, 44.4203) ccw
  arc A33 (133.315, 45.904) -> (135.5431, 44.9065) centre (135.0765, 46.8513) ccw
  arc A34 (134.4566, 48.0619) -> (133.315, 45.904) centre (135.2862, 46.2421) ccw
  arc A35 (134.4566, 48.0619) -> (134.719, 48.6879) centre (134.2492, 48.5169) ccw
  line L9 (134.719, 48.6879) -> (134.4967, 49.2987)
  arc A36 (134.4967, 49.2987) -> (133.8933, 49.6095) centre (134.0269, 49.1277) ccw
  arc A37 (131.6318, 50.5287) -> (133.8933, 49.6095) centre (133.3591, 51.5368) ccw
  arc A38 (132.6974, 52.7251) -> (131.6318, 50.5287) centre (133.59, 50.9353) ccw
  arc A39 (132.6974, 52.7251) -> (132.9378, 53.3598) centre (132.4742, 53.1725) ccw
  line L10 (132.9378, 53.3598) -> (132.6943, 53.9625)
  arc A40 (132.6943, 53.9625) -> (132.0804, 54.2521) centre (132.2307, 53.7752) ccw
  arc A41 (129.7882, 55.0918) -> (132.0804, 54.2521) centre (131.4793, 56.1596) ccw
  arc A42 (130.7764, 57.324) -> (129.7882, 55.0918) centre (131.731, 55.5665) ccw
  arc A43 (130.7764, 57.324) -> (130.9946, 57.9668) centre (130.5378, 57.7634) ccw
  line L11 (130.9946, 57.9668) -> (130.7302, 58.5606)
  arc A44 (130.7302, 58.5606) -> (130.1066, 58.8286) centre (130.2734, 58.3572) ccw
  arc A45 (127.7864, 59.5878) -> (130.1066, 58.8286) centre (129.4392, 60.7139) ccw
  arc A46 (128.6962, 61.8532) -> (127.7864, 59.5878) centre (129.7115, 60.13) ccw
  arc A47 (128.6962, 61.8532) -> (128.8918, 62.5031) centre (128.4424, 62.2839) ccw
  line L12 (128.8918, 62.5031) -> (128.6068, 63.0873)
  arc A48 (128.6068, 63.0873) -> (127.9742, 63.3334) centre (128.1574, 62.8682) ccw
  arc A49 (125.629, 64.0112) -> (127.9742, 63.3334) centre (127.2415, 65.1943) ccw
  arc A50 (126.4592, 66.3069) -> (125.629, 64.0112) centre (127.534, 64.6203) ccw
  arc A51 (126.4592, 66.3069) -> (126.6319, 66.9633) centre (126.1905, 66.7286) ccw
  line L13 (126.6319, 66.9633) -> (126.3268, 67.5372)
  arc A52 (126.3268, 67.5372) -> (125.686, 67.761) centre (125.8853, 67.3025) ccw
  arc A53 (123.3185, 68.3566) -> (125.686, 67.761) centre (124.8887, 69.5953) ccw
  arc A54 (124.068, 70.6799) -> (123.3185, 68.3566) centre (125.2011, 69.0318) ccw
  arc A55 (124.068, 70.6799) -> (124.2178, 71.3419) centre (123.7848, 71.0919) ccw
  line L14 (124.2178, 71.3419) -> (123.8928, 71.9048)
  arc A56 (123.8928, 71.9048) -> (123.2446, 72.1061) centre (123.4598, 71.6548) ccw
  arc A57 (120.8578, 72.6187) -> (123.2446, 72.1061) centre (122.3838, 73.9114) ccw
  arc A58 (121.5258, 74.9667) -> (120.8578, 72.6187) centre (122.7156, 73.3592) ccw
  arc A59 (121.5258, 74.9667) -> (121.6523, 75.6336) centre (121.2283, 75.3686) ccw
  line L15 (121.6523, 75.6336) -> (121.3079, 76.1848)
  arc A60 (121.3079, 76.1848) -> (120.653, 76.3634) centre (120.8839, 75.9199) ccw
  arc A61 (118.2498, 76.7923) -> (120.653, 76.3634) centre (119.7298, 78.1375) ccw
  arc A62 (118.8354, 79.1623) -> (118.2498, 76.7923) centre (120.0807, 77.5972) ccw
  arc A63 (118.8354, 79.1623) -> (118.9387, 79.8331) centre (118.5241, 79.5535) ccw
  line L16 (118.9387, 79.8331) -> (118.5752, 80.372)
  arc A64 (118.5752, 80.372) -> (117.9145, 80.5276) centre (118.1607, 80.0924) ccw
  arc A65 (115.4978, 80.8724) -> (117.9145, 80.5276) centre (116.9299, 82.2684) ccw
  arc A66 (116.0003, 83.2613) -> (115.4978, 80.8724) centre (117.2994, 81.7407) ccw
  arc A67 (116.0003, 83.2613) -> (116.0801, 83.9354) centre (115.6756, 83.6415) ccw
  line L17 (116.0801, 83.9354) -> (115.698, 84.4612)
  arc A68 (115.698, 84.4612) -> (115.0323, 84.5937) centre (115.2935, 84.1673) ccw
  arc A69 (112.605, 84.8539) -> (115.0323, 84.5937) centre (113.9875, 86.2991) ccw
  arc A70 (113.0239, 87.259) -> (112.605, 84.8539) centre (114.3753, 85.7846) ccw
  arc A71 (113.0239, 87.259) -> (113.08, 87.9354) centre (112.686, 87.6276) ccw
  line L18 (113.08, 87.9354) -> (112.6799, 88.4476)
  arc A72 (112.6799, 88.4476) -> (112.01, 88.5567) centre (112.2859, 88.1398) ccw
  arc A73 (109.575, 88.7321) -> (112.01, 88.5567) centre (110.9063, 90.2247) ccw
  arc A74 (109.9097, 91.1503) -> (109.575, 88.7321) centre (111.3118, 89.724) ccw
  arc A75 (109.9097, 91.1503) -> (109.9423, 91.8283) centre (109.5592, 91.5069) ccw
  line L19 (109.9423, 91.8283) -> (109.5244, 92.3262)
  arc A76 (109.5244, 92.3262) -> (108.8511, 92.4119) centre (109.1414, 92.0048) ccw
  arc A77 (106.4116, 92.5022) -> (108.8511, 92.4119) centre (107.6899, 94.0403) ccw
  arc A78 (106.6617, 94.9306) -> (106.4116, 92.5022) centre (108.1126, 93.554) ccw
  arc A79 (106.6617, 94.9306) -> (106.6705, 95.6092) centre (106.299, 95.2747) ccw
  line L20 (106.6705, 95.6092) -> (106.2356, 96.0923)
  arc A80 (106.2356, 96.0923) -> (105.5597, 96.1544) centre (105.864, 95.7577) ccw
  arc A81 (103.1185, 96.1595) -> (105.5597, 96.1544) centre (104.3424, 97.7413) ccw
  arc A82 (103.2837, 98.5952) -> (103.1185, 96.1595) centre (104.7818, 97.2701) ccw
  arc A83 (103.2837, 98.5952) -> (103.2688, 99.2737) centre (102.9092, 98.9264) ccw
  line L21 (103.2688, 99.2737) -> (102.8173, 99.7413)
  arc A84 (102.8173, 99.7413) -> (102.1396, 99.7798) centre (102.4576, 99.394) ccw
  arc A85 (99.6997, 99.6997) -> (102.1396, 99.7798) centre (100.8677, 101.3233) ccw
  arc A86 (99.7798, 102.1396) -> (99.6997, 99.6997) centre (101.3233, 100.8677) ccw
  arc A87 (99.7798, 102.1396) -> (99.7413, 102.8173) centre (99.394, 102.4576) ccw
  line L22 (99.7413, 102.8173) -> (99.2737, 103.2688)
  arc A88 (99.2737, 103.2688) -> (98.5952, 103.2837) centre (98.9264, 102.9092) ccw
  arc A89 (96.1595, 103.1185) -> (98.5952, 103.2837) centre (97.2701, 104.7818) ccw
  arc A90 (96.1544, 105.5597) -> (96.1595, 103.1185) centre (97.7413, 104.3424) ccw
  arc A91 (96.1544, 105.5597) -> (96.0923, 106.2356) centre (95.7577, 105.864) ccw
  line L23 (96.0923, 106.2356) -> (95.6092, 106.6705)
  arc A92 (95.6092, 106.6705) -> (94.9306, 106.6617) centre (95.2747, 106.299) ccw
  arc A93 (92.5022, 106.4116) -> (94.9306, 106.6617) centre (93.554, 108.1126) ccw
  arc A94 (92.4119, 108.8511) -> (92.5022, 106.4116) centre (94.0403, 107.6899) ccw
  arc A95 (92.4119, 108.8511) -> (92.3262, 109.5244) centre (92.0048, 109.1414) ccw
  line L24 (92.3262, 109.5244) -> (91.8283, 109.9423)
  arc A96 (91.8283, 109.9423) -> (91.1503, 109.9097) centre (91.5069, 109.5592) ccw
  arc A97 (88.7321, 109.575) -> (91.1503, 109.9097) centre (89.724, 111.3118) ccw
  arc A98 (88.5567, 112.01) -> (88.7321, 109.575) centre (90.2247, 110.9063) ccw
  arc A99 (88.5567, 112.01) -> (88.4476, 112.6799) centre (88.1398, 112.2859) ccw
  line L25 (88.4476, 112.6799) -> (87.9354, 113.08)
  arc A100 (87.9354, 113.08) -> (87.259, 113.0239) centre (87.6276, 112.686) ccw
  arc A101 (84.8539, 112.605) -> (87.259, 113.0239) centre (85.7846, 114.3753) ccw
  arc A102 (84.5937, 115.0323) -> (84.8539, 112.605) centre (86.2991, 113.9875) ccw
  arc A103 (84.5937, 115.0323) -> (84.4612, 115.698) centre (84.1673, 115.2935) ccw
  line L26 (84.4612, 115.698) -> (83.9354, 116.0801)
  arc A104 (83.9354, 116.0801) -> (83.2613, 116.0003) centre (83.6415, 115.6756) ccw
  arc A105 (80.8724, 115.4978) -> (83.2613, 116.0003) centre (81.7407, 117.2994) ccw
  arc A106 (80.5276, 117.9145) -> (80.8724, 115.4978) centre (82.2684, 116.9299) ccw
  arc A107 (80.5276, 117.9145) -> (80.372, 118.5752) centre (80.0924, 118.1607) ccw
  line L27 (80.372, 118.5752) -> (79.8331, 118.9387)
  arc A108 (79.8331, 118.9387) -> (79.1623, 118.8354) centre (79.5535, 118.5241) ccw
  arc A109 (76.7923, 118.2498) -> (79.1623, 118.8354) centre (77.5972, 120.0807) ccw
  arc A110 (76.3634, 120.653) -> (76.7923, 118.2498) centre (78.1375, 119.7298) ccw
  arc A111 (76.3634, 120.653) -> (76.1848, 121.3079) centre (75.9199, 120.8839) ccw
  line L28 (76.1848, 121.3079) -> (75.6336, 121.6523)
  arc A112 (75.6336, 121.6523) -> (74.9667, 121.5258) centre (75.3686, 121.2283) ccw
  arc A113 (72.6187, 120.8578) -> (74.9667, 121.5258) centre (73.3592, 122.7156) ccw
  arc A114 (72.1061, 123.2446) -> (72.6187, 120.8578) centre (73.9114, 122.3838) ccw
  arc A115 (72.1061, 123.2446) -> (71.9048, 123.8928) centre (71.6548, 123.4598) ccw
  line L29 (71.9048, 123.8928) -> (71.3419, 124.2178)
  arc A116 (71.3419, 124.2178) -> (70.6799, 124.068) centre (71.0919, 123.7848) ccw
  arc A117 (68.3566, 123.3185) -> (70.6799, 124.068) centre (69.0318, 125.2011) ccw
  arc A118 (67.761, 125.686) -> (68.3566, 123.3185) centre (69.5953, 124.8887) ccw
  arc A119 (67.761, 125.686) -> (67.5372, 126.3268) centre (67.3025, 125.8853) ccw
  line L30 (67.5372, 126.3268) -> (66.9633, 126.6319)
  arc A120 (66.9633, 126.6319) -> (66.3069, 126.4592) centre (66.7286, 126.1905) ccw
  arc A121 (64.0112, 125.629) -> (66.3069, 126.4592) centre (64.6203, 127.534) ccw
  arc A122 (63.3334, 127.9742) -> (64.0112, 125.629) centre (65.1943, 127.2415) ccw
  arc A123 (63.3334, 127.9742) -> (63.0873, 128.6068) centre (62.8682, 128.1574) ccw
  line L31 (63.0873, 128.6068) -> (62.5031, 128.8918)
  arc A124 (62.5031, 128.8918) -> (61.8532, 128.6962) centre (62.2839, 128.4424) ccw
  arc A125 (59.5878, 127.7864) -> (61.8532, 128.6962) centre (60.13, 129.7115) ccw
  arc A126 (58.8286, 130.1066) -> (59.5878, 127.7864) centre (60.7139, 129.4392) ccw
  arc A127 (58.8286, 130.1066) -> (58.5606, 130.7302) centre (58.3572, 130.2734) ccw
  line L32 (58.5606, 130.7302) -> (57.9668, 130.9946)
  arc A128 (57.9668, 130.9946) -> (57.324, 130.7764) centre (57.7634, 130.5378) ccw
  arc A129 (55.0918, 129.7882) -> (57.324, 130.7764) centre (55.5665, 131.731) ccw
  arc A130 (54.2521, 132.0804) -> (55.0918, 129.7882) centre (56.1596, 131.4793) ccw
  arc A131 (54.2521, 132.0804) -> (53.9625, 132.6943) centre (53.7752, 132.2307) ccw
  line L33 (53.9625, 132.6943) -> (53.3598, 132.9378)
  arc A132 (53.3598, 132.9378) -> (52.7251, 132.6974) centre (53.1725, 132.4742) ccw
  arc A133 (50.5287, 131.6318) -> (52.7251, 132.6974) centre (50.9353, 133.59) ccw
  arc A134 (49.6095, 133.8933) -> (50.5287, 131.6318) centre (51.5368, 133.3591) ccw
  arc A135 (49.6095, 133.8933) -> (49.2987, 134.4967) centre (49.1277, 134.0269) ccw
  line L34 (49.2987, 134.4967) -> (48.6879, 134.719)
  arc A136 (48.6879, 134.719) -> (48.0619, 134.4566) centre (48.5169, 134.2492) ccw
  arc A137 (45.904, 133.315) -> (48.0619, 134.4566) centre (46.2421, 135.2862) ccw
  arc A138 (44.9065, 135.5431) -> (45.904, 133.315) centre (46.8513, 135.0765) ccw
  arc A139 (44.9065, 135.5431) -> (44.5748, 136.1353) centre (44.4203, 135.6598) ccw
  line L35 (44.5748, 136.1353) -> (43.9566, 136.3362)
  arc A140 (43.9566, 136.3362) -> (43.3402, 136.052) centre (43.8021, 135.8606) ccw
  arc A141 (41.2235, 134.8358) -> (43.3402, 136.052) centre (41.4925, 136.8177) ccw
  arc A142 (40.1487, 137.0278) -> (41.2235, 134.8358) centre (42.1086, 136.6293) ccw
  arc A143 (40.1487, 137.0278) -> (39.7966, 137.608) centre (39.6587, 137.1274) ccw
  line L36 (39.7966, 137.608) -> (39.1717, 137.7872)
  arc A144 (39.1717, 137.7872) -> (38.5656, 137.4817) centre (39.0339, 137.3065) ccw
  arc A145 (36.4926, 136.1924) -> (38.5656, 137.4817) centre (36.6924, 138.1824) ccw
  arc A146 (35.3421, 138.3455) -> (36.4926, 136.1924) centre (37.3147, 138.0156) ccw
  arc A147 (35.3421, 138.3455) -> (34.9699, 138.9131) centre (34.8489, 138.4279) ccw
  line L37 (34.9699, 138.9131) -> (34.3392, 139.0703)
  arc A148 (34.3392, 139.0703) -> (33.7441, 138.7439) centre (34.2182, 138.5852) ccw
  arc A149 (31.7174, 137.383) -> (33.7441, 138.7439) centre (31.8475, 139.3787) ccw
  arc A150 (30.4923, 139.4946) -> (31.7174, 137.383) centre (32.4753, 139.2338) ccw
  arc A151 (30.4923, 139.4946) -> (30.1006, 140.0489) centre (29.9966, 139.5598) ccw
  line L38 (30.1006, 140.0489) -> (29.4648, 140.184)
  arc A152 (29.4648, 140.184) -> (28.8814, 139.837) centre (29.3608, 139.6949) ccw
  arc A153 (26.9034, 138.4062) -> (28.8814, 139.837) centre (26.9639, 140.4053) ccw
  arc A154 (25.6055, 140.4738) -> (26.9034, 138.4062) centre (27.5963, 140.2824) ccw
  arc A155 (25.6055, 140.4738) -> (25.1946, 141.014) centre (25.1078, 140.5216) ccw
  line L39 (25.1946, 141.014) -> (24.5545, 141.1269)
  arc A156 (24.5545, 141.1269) -> (23.9836, 140.7598) centre (24.4676, 140.6345) ccw
  arc A157 (22.0567, 139.2608) -> (23.9836, 140.7598) centre (22.0474, 141.2608) ccw
  arc A158 (20.6874, 141.2818) -> (22.0567, 139.2608) centre (22.6837, 141.16) ccw
  arc A159 (20.6874, 141.2818) -> (20.2579, 141.8074) centre (20.1883, 141.3123) ccw
  line L40 (20.2579, 141.8074) -> (19.6143, 141.8979)
  arc A160 (19.6143, 141.8979) -> (19.0565, 141.511) centre (19.5447, 141.4028) ccw
  arc A161 (17.1832, 139.9458) -> (19.0565, 141.511) centre (17.104, 141.9442) ccw
  arc A162 (15.7441, 141.9177) -> (17.1832, 139.9458) centre (17.7435, 141.8657) ccw
  arc A163 (15.7441, 141.9177) -> (15.2966, 142.428) centre (15.2443, 141.9308) ccw
  line L41 (15.2966, 142.428) -> (14.6501, 142.496)
  arc A164 (14.6501, 142.496) -> (14.1063, 142.0899) centre (14.5979, 141.9987) ccw
  arc A165 (12.2887, 140.4602) -> (14.1063, 142.0899) centre (12.1398, 142.4546) ccw
  arc A166 (10.7817, 142.3808) -> (12.2887, 140.4602) centre (12.7816, 142.3985) ccw
  arc A167 (10.7817, 142.3808) -> (10.3166, 142.8751) centre (10.2817, 142.3763) ccw
  line L42 (10.3166, 142.8751) -> (9.6682, 142.9205)
  arc A168 (9.6682, 142.9205) -> (9.1388, 142.4956) centre (9.6333, 142.4217) ccw
  arc A169 (7.3792, 140.8035) -> (9.1388, 142.4956) centre (7.1608, 142.7915) ccw
  arc A170 (5.8061, 142.6703) -> (7.3792, 140.8035) centre (7.8042, 142.7578) ccw
  arc A171 (5.8061, 142.6703) -> (5.324, 143.1481) centre (5.3066, 142.6484) ccw
  line L43 (5.324, 143.1481) -> (4.6744, 143.1708)
  arc A172 (4.6744, 143.1708) -> (4.1602, 142.7278) centre (4.657, 142.6711) ccw
  arc A173 (2.4607, 140.9752) -> (4.1602, 142.7278) centre (2.1731, 142.9545) ccw
  arc A174 (0.8235, 142.786) -> (2.4607, 140.9752) centre (2.8173, 142.9432) ccw
  arc A175 (0.8235, 142.786) -> (0.325, 143.2467) centre (0.325, 142.7467) ccw
  line L44 (0.325, 143.2467) -> (-0.325, 143.2467)
  arc A176 (-0.325, 143.2467) -> (-0.8235, 142.786) centre (-0.325, 142.7467) ccw
  arc A177 (-2.4607, 140.9752) -> (-0.8235, 142.786) centre (-2.8173, 142.9432) ccw
  arc A178 (-4.1602, 142.7278) -> (-2.4607, 140.9752) centre (-2.1731, 142.9545) ccw
  arc A179 (-4.1602, 142.7278) -> (-4.6744, 143.1708) centre (-4.657, 142.6711) ccw
  line L45 (-4.6744, 143.1708) -> (-5.324, 143.1481)
  arc A180 (-5.324, 143.1481) -> (-5.8061, 142.6703) centre (-5.3066, 142.6484) ccw
  arc A181 (-7.3792, 140.8035) -> (-5.8061, 142.6703) centre (-7.8042, 142.7578) ccw
  arc A182 (-9.1388, 142.4956) -> (-7.3792, 140.8035) centre (-7.1608, 142.7915) ccw
  arc A183 (-9.1388, 142.4956) -> (-9.6682, 142.9205) centre (-9.6333, 142.4217) ccw
  line L46 (-9.6682, 142.9205) -> (-10.3166, 142.8751)
  arc A184 (-10.3166, 142.8751) -> (-10.7817, 142.3808) centre (-10.2817, 142.3763) ccw
  arc A185 (-12.2887, 140.4602) -> (-10.7817, 142.3808) centre (-12.7816, 142.3985) ccw
  arc A186 (-14.1063, 142.0899) -> (-12.2887, 140.4602) centre (-12.1398, 142.4546) ccw
  arc A187 (-14.1063, 142.0899) -> (-14.6501, 142.496) centre (-14.5979, 141.9987) ccw
  line L47 (-14.6501, 142.496) -> (-15.2966, 142.428)
  arc A188 (-15.2966, 142.428) -> (-15.7441, 141.9177) centre (-15.2443, 141.9308) ccw
  arc A189 (-17.1832, 139.9458) -> (-15.7441, 141.9177) centre (-17.7435, 141.8657) ccw
  arc A190 (-19.0565, 141.511) -> (-17.1832, 139.9458) centre (-17.104, 141.9442) ccw
  arc A191 (-19.0565, 141.511) -> (-19.6143, 141.8979) centre (-19.5447, 141.4028) ccw
  line L48 (-19.6143, 141.8979) -> (-20.2579, 141.8074)
  arc A192 (-20.2579, 141.8074) -> (-20.6874, 141.2818) centre (-20.1883, 141.3123) ccw
  arc A193 (-22.0567, 139.2608) -> (-20.6874, 141.2818) centre (-22.6837, 141.16) ccw
  arc A194 (-23.9836, 140.7598) -> (-22.0567, 139.2608) centre (-22.0474, 141.2608) ccw
  arc A195 (-23.9836, 140.7598) -> (-24.5545, 141.1269) centre (-24.4676, 140.6345) ccw
  line L49 (-24.5545, 141.1269) -> (-25.1946, 141.014)
  arc A196 (-25.1946, 141.014) -> (-25.6055, 140.4738) centre (-25.1078, 140.5216) ccw
  arc A197 (-26.9034, 138.4062) -> (-25.6055, 140.4738) centre (-27.5963, 140.2824) ccw
  arc A198 (-28.8814, 139.837) -> (-26.9034, 138.4062) centre (-26.9639, 140.4053) ccw
  arc A199 (-28.8814, 139.837) -> (-29.4648, 140.184) centre (-29.3608, 139.6949) ccw
  line L50 (-29.4648, 140.184) -> (-30.1006, 140.0489)
  arc A200 (-30.1006, 140.0489) -> (-30.4923, 139.4946) centre (-29.9966, 139.5598) ccw
  arc A201 (-31.7174, 137.383) -> (-30.4923, 139.4946) centre (-32.4753, 139.2338) ccw
  arc A202 (-33.7441, 138.7439) -> (-31.7174, 137.383) centre (-31.8475, 139.3787) ccw
  arc A203 (-33.7441, 138.7439) -> (-34.3392, 139.0703) centre (-34.2182, 138.5852) ccw
  line L51 (-34.3392, 139.0703) -> (-34.9699, 138.9131)
  arc A204 (-34.9699, 138.9131) -> (-35.3421, 138.3455) centre (-34.8489, 138.4279) ccw
  arc A205 (-36.4926, 136.1924) -> (-35.3421, 138.3455) centre (-37.3147, 138.0156) ccw
  arc A206 (-38.5656, 137.4817) -> (-36.4926, 136.1924) centre (-36.6924, 138.1824) ccw
  arc A207 (-38.5656, 137.4817) -> (-39.1717, 137.7872) centre (-39.0339, 137.3065) ccw
  line L52 (-39.1717, 137.7872) -> (-39.7966, 137.608)
  arc A208 (-39.7966, 137.608) -> (-40.1487, 137.0278) centre (-39.6587, 137.1274) ccw
  arc A209 (-41.2235, 134.8358) -> (-40.1487, 137.0278) centre (-42.1086, 136.6293) ccw
  arc A210 (-43.3402, 136.052) -> (-41.2235, 134.8358) centre (-41.4925, 136.8177) ccw
  arc A211 (-43.3402, 136.052) -> (-43.9566, 136.3362) centre (-43.8021, 135.8606) ccw
  line L53 (-43.9566, 136.3362) -> (-44.5748, 136.1353)
  arc A212 (-44.5748, 136.1353) -> (-44.9065, 135.5431) centre (-44.4203, 135.6598) ccw
  arc A213 (-45.904, 133.315) -> (-44.9065, 135.5431) centre (-46.8513, 135.0765) ccw
  arc A214 (-48.0619, 134.4566) -> (-45.904, 133.315) centre (-46.2421, 135.2862) ccw
  arc A215 (-48.0619, 134.4566) -> (-48.6879, 134.719) centre (-48.5169, 134.2492) ccw
  line L54 (-48.6879, 134.719) -> (-49.2987, 134.4967)
  arc A216 (-49.2987, 134.4967) -> (-49.6095, 133.8933) centre (-49.1277, 134.0269) ccw
  arc A217 (-50.5287, 131.6318) -> (-49.6095, 133.8933) centre (-51.5368, 133.3591) ccw
  arc A218 (-52.7251, 132.6974) -> (-50.5287, 131.6318) centre (-50.9353, 133.59) ccw
  arc A219 (-52.7251, 132.6974) -> (-53.3598, 132.9378) centre (-53.1725, 132.4742) ccw
  line L55 (-53.3598, 132.9378) -> (-53.9625, 132.6943)
  arc A220 (-53.9625, 132.6943) -> (-54.2521, 132.0804) centre (-53.7752, 132.2307) ccw
  arc A221 (-55.0918, 129.7882) -> (-54.2521, 132.0804) centre (-56.1596, 131.4793) ccw
  arc A222 (-57.324, 130.7764) -> (-55.0918, 129.7882) centre (-55.5665, 131.731) ccw
  arc A223 (-57.324, 130.7764) -> (-57.9668, 130.9946) centre (-57.7634, 130.5378) ccw
  line L56 (-57.9668, 130.9946) -> (-58.5606, 130.7302)
  arc A224 (-58.5606, 130.7302) -> (-58.8286, 130.1066) centre (-58.3572, 130.2734) ccw
  arc A225 (-59.5878, 127.7864) -> (-58.8286, 130.1066) centre (-60.7139, 129.4392) ccw
  arc A226 (-61.8532, 128.6962) -> (-59.5878, 127.7864) centre (-60.13, 129.7115) ccw
  arc A227 (-61.8532, 128.6962) -> (-62.5031, 128.8918) centre (-62.2839, 128.4424) ccw
  line L57 (-62.5031, 128.8918) -> (-63.0873, 128.6068)
  arc A228 (-63.0873, 128.6068) -> (-63.3334, 127.9742) centre (-62.8682, 128.1574) ccw
  arc A229 (-64.0112, 125.629) -> (-63.3334, 127.9742) centre (-65.1943, 127.2415) ccw
  arc A230 (-66.3069, 126.4592) -> (-64.0112, 125.629) centre (-64.6203, 127.534) ccw